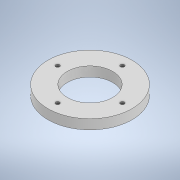
# Autodesk Inventor part: horizontal_lower_bearing_holder
Saved by Autodesk Inventor 2021 (Build 250183000, 183)
## iProperties
Created: 2020-10-10
Part Number: horizontal_lower_bearing_holder
Material: Generic
Document SubType Name: Modeling
Designer: bober
Density: 1 g/cm^3
Appearance: Default
Author: bober
Autodesk Inventor part; units mm, degrees
ref_plane "YZ Plane" through (0, 0, 0) normal (1, 0, 0) x (0, 1, 0)
ref_plane "XZ Plane" through (0, 0, 0) normal (0, 1, 0) x (-1, 0, 0)
ref_plane "XY Plane" through (0, 0, 0) normal (0, 0, 1) x (1, 0, 0)
sketch "Sketch1" plane through (0, 0, 0) normal (0, 1, 0) x (-1, 0, 0)
  circle A0 centre (0, 0) radius 23.5
  circle A1 centre (0, 0) radius 43.5
  dimension "d0" = 47
  dimension "d1" = 87
  constraints: 2 centre point, 2 coincident
  measures "d0" diameter of A0
  measures "d1" diameter of A1
extrude "Extrusion1" add sketch "Sketch1" along normal blind 10
sketch "Sketch2" plane through (0, 10, 0) normal (0, 1, 0) x (1, 0, 0)
  circle A0 centre (33.5, 0) radius 2
  point P0 (0, 0)
  dimension "d4" = 4
  constraints: 1 centre point
  measures "d4" diameter of A0
extrude "Extrusion2" cut sketch "Sketch2" against normal blind 10
mirror "Mirror1" about plane through (0, 0, 0) normal (1, 0, 0) of "Extrusion2"
sketch "Sketch3" plane through (0, 10, 0) normal (0, 1, 0) x (1, 0, 0)
  circle A0 centre (0, 33.5) radius 2
  circle A1 centre (0, -33.5) radius 2
  point P0 (0, 0)
  dimension "d7" = 4
  dimension "d8" = 4
  constraints: 2 centre point
  measures "d7" diameter of A0
  measures "d8" diameter of A1
extrude "Extrusion3" cut sketch "Sketch3" against normal blind 10
body "Solid1"
